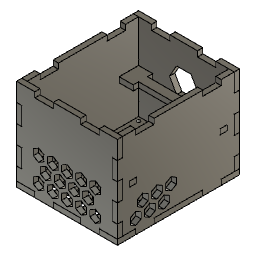
case (Autodesk Fusion 360 design; units mm, degrees)
Autodesk Fusion 360 part; units mm, degrees
(part 1 of 2)
ref_plane "WorkPlane4" through (0, 0, -25.9) normal (0, 0, 1) x (1, 0, 0)
sketch "Bottom" plane through (0, 0, -25.9) normal (0, 0, 1) x (1, 0, 0)
  line L0 (28.5, -34.5) -> (-28.5, -34.5)
  line L1 (-28.5, -34.5) -> (-28.5, 34.5)
  line L2 (-28.5, 34.5) -> (28.5, 34.5)
  line L3 (28.5, 34.5) -> (28.5, -34.5)
  line L4 (28.5, -34.5) -> (-28.5, 34.5) construction
  line L5 (-28.5, -34.5) -> (28.5, 34.5) construction
  line L6 (-18.14, 34.5) -> (-7.78, 34.5)
  line L7 (-7.78, 34.5) -> (-7.78, 31.5)
  line L8 (-7.78, 31.5) -> (-18.14, 31.5)
  line L9 (-18.14, 31.5) -> (-18.14, 34.5)
  line L10 (-28.5, 49.5405) -> (-18.14, 49.5405) construction
  line L11 (-28.5, 24.14) -> (-25.5, 24.14)
  line L12 (-25.5, 24.14) -> (-25.5, 13.78)
  line L13 (-25.5, 13.78) -> (-28.5, 13.78)
  line L14 (-28.5, 13.78) -> (-28.5, 24.14)
  line L15 (-32.8454, 24.14) -> (-32.8454, 34.5) construction
  line L16 (0, 34.5) -> (0, -34.5) construction
  line L17 (7.78, 34.5) -> (7.78, 31.5)
  line L18 (28.5, 49.5405) -> (18.14, 49.5405) construction
  line L19 (7.78, 31.5) -> (18.14, 31.5)
  line L20 (18.14, 31.5) -> (18.14, 34.5)
  line L21 (18.14, 34.5) -> (7.78, 34.5)
  line L22 (-28.5, 0) -> (28.5, 0) construction
  line L23 (-28.5, -24.14) -> (-25.5, -24.14)
  line L24 (-28.5, -13.78) -> (-28.5, -24.14)
  line L25 (-25.5, -24.14) -> (-25.5, -13.78)
  line L26 (-25.5, -13.78) -> (-28.5, -13.78)
  line L27 (-32.8454, -24.14) -> (-32.8454, -34.5) construction
  line L28 (28.5, 13.78) -> (28.5, 24.14)
  line L29 (28.5, -13.78) -> (28.5, -24.14)
  line L30 (25.5, 13.78) -> (28.5, 13.78)
  line L31 (28.5, 24.14) -> (25.5, 24.14)
  line L32 (32.8454, 24.14) -> (32.8454, 34.5) construction
  line L33 (28.5, -24.14) -> (25.5, -24.14)
  line L34 (25.5, -24.14) -> (25.5, -13.78)
  line L35 (32.8454, -24.14) -> (32.8454, -34.5) construction
  line L36 (25.5, -13.78) -> (28.5, -13.78)
  line L37 (25.5, 24.14) -> (25.5, 13.78)
  line L38 (-7.78, -31.5) -> (-18.14, -31.5)
  line L39 (7.78, -31.5) -> (18.14, -31.5)
  line L40 (18.14, -31.5) -> (18.14, -34.5)
  line L41 (18.14, -34.5) -> (7.78, -34.5)
  line L42 (-18.14, -34.5) -> (-7.78, -34.5)
  line L43 (28.5, -49.5405) -> (18.14, -49.5405) construction
  line L44 (7.78, -34.5) -> (7.78, -31.5)
  line L45 (-7.78, -34.5) -> (-7.78, -31.5)
  line L46 (-28.5, -49.5405) -> (-18.14, -49.5405) construction
  line L47 (-18.14, -31.5) -> (-18.14, -34.5)
  line L48 (-28.5, 34.5) -> (-23.32, 34.5) construction
  line L49 (-23.32, 34.5) -> (-23.32, 29.32) construction
  line L50 (-23.32, 29.32) -> (-28.5, 29.32) construction
  line L51 (-28.5, 29.32) -> (-28.5, 34.5) construction
  circle A0 centre (-23.32, 29.32) radius 1
  line L52 (-28.5, -34.5) -> (-23.32, -34.5) construction
  line L53 (-23.32, -34.5) -> (-23.32, -29.32) construction
  line L54 (-23.32, -29.32) -> (-28.5, -29.32) construction
  line L55 (-28.5, -29.32) -> (-28.5, -34.5) construction
  circle A1 centre (-23.32, -29.32) radius 1
  line L56 (28.5, -34.5) -> (23.32, -34.5) construction
  line L57 (23.32, -34.5) -> (23.32, -29.32) construction
  line L58 (23.32, -29.32) -> (28.5, -29.32) construction
  line L59 (28.5, -29.32) -> (28.5, -34.5) construction
  line L60 (28.5, 34.5) -> (23.32, 34.5) construction
  line L61 (23.32, 34.5) -> (23.32, 29.32) construction
  line L62 (23.32, 29.32) -> (28.5, 29.32) construction
  line L63 (28.5, 29.32) -> (28.5, 34.5) construction
  circle A2 centre (23.32, -29.32) radius 1
  circle A3 centre (23.32, 29.32) radius 1
  line L64 (0, -26.5) -> (-28.5, -26.5) construction
  line L65 (-13, -24.7679) -> (-16, -23.0359)
  line L66 (-1, -17.8397) -> (-4, -16.1077)
  line L67 (5, -24.7679) -> (5, -28.2321)
  line L68 (-3, -10.9115) -> (-3, -14.3756)
  line L69 (0, -26.5) -> (-1.5, -23.9019) construction
  line L70 (3, -28.2321) -> (3, -24.7679)
  line L71 (9, -21.3038) -> (12, -23.0359)
  line L72 (-11, -24.7679) -> (-11, -28.2321)
  line L73 (13, -14.3756) -> (16, -16.1077)
  line L74 (7, -21.3038) -> (7, -17.8397)
  line L75 (15, -21.3038) -> (15, -17.8397)
  line L76 (-16, -29.9641) -> (-13, -28.2321)
  line L77 (13, -28.2321) -> (16, -29.9641)
  line L78 (8, -9.1795) -> (5, -10.9115)
  line L79 (5, -14.3756) -> (8, -16.1077)
  line L80 (-19, -28.2321) -> (-16, -29.9641)
  line L81 (1, -17.8397) -> (1, -21.3038)
  line L82 (-13, -28.2321) -> (-13, -24.7679)
  line L83 (-13, -14.3756) -> (-13, -10.9115)
  line L84 (-11, -10.9115) -> (-11, -14.3756)
  line L85 (-4, -16.1077) -> (-7, -17.8397)
  line L86 (-5, -14.3756) -> (-5, -10.9115)
  line L87 (-8, -9.1795) -> (-11, -10.9115)
  line L88 (-3, -24.7679) -> (-3, -28.2321)
  line L89 (-8, -16.1077) -> (-5, -14.3756)
  line L90 (19, -28.2321) -> (19, -24.7679)
  line L91 (-19, -14.3756) -> (-16, -16.1077)
  line L92 (15, -17.8397) -> (12, -16.1077)
  line L93 (-19, -24.7679) -> (-19, -28.2321)
  line L94 (16, -29.9641) -> (19, -28.2321)
  line L95 (8, -29.9641) -> (11, -28.2321)
  line L96 (1, -21.3038) -> (4, -23.0359)
  line L97 (16, -16.1077) -> (19, -14.3756)
  line L98 (-12, -23.0359) -> (-9, -21.3038)
  line L99 (-4, -23.0359) -> (-1, -21.3038)
  line L100 (-11, -14.3756) -> (-8, -16.1077)
  line L101 (19, -14.3756) -> (19, -10.9115)
  line L102 (7, -17.8397) -> (4, -16.1077)
  line L103 (12, -16.1077) -> (9, -17.8397)
  line L104 (4, -23.0359) -> (7, -21.3038)
  line L105 (13, -10.9115) -> (13, -14.3756)
  line L106 (8, -23.0359) -> (5, -24.7679)
  line L107 (-5, -28.2321) -> (-5, -24.7679)
  line L108 (-16, -16.1077) -> (-13, -14.3756)
  line L109 (11, -14.3756) -> (11, -10.9115)
  line L110 (-7, -21.3038) -> (-4, -23.0359)
  line L111 (-5, -10.9115) -> (-8, -9.1795)
  line L112 (-3, -14.3756) -> (0, -16.1077)
  line L113 (-13, -10.9115) -> (-16, -9.1795)
  line L114 (3, -14.3756) -> (3, -10.9115)
  line L115 (-15, -21.3038) -> (-12, -23.0359)
  line L116 (-1, -21.3038) -> (-1, -17.8397)
  line L117 (19, -10.9115) -> (16, -9.1795)
  line L118 (-7, -17.8397) -> (-7, -21.3038)
  line L119 (0, -34.5) -> (0, -26.5) construction
  line L120 (-3, -28.2321) -> (0, -29.9641)
  line L121 (12, -23.0359) -> (15, -21.3038)
  line L122 (-15, -17.8397) -> (-15, -21.3038)
  line L123 (-28.5, -26.5) -> (-28.5, -34.5) construction
  line L124 (4, -16.1077) -> (1, -17.8397)
  line L125 (11, -28.2321) -> (11, -24.7679)
  line L126 (8, -16.1077) -> (11, -14.3756)
  line L127 (3, -10.9115) -> (0, -9.1795)
  line L128 (9, -17.8397) -> (9, -21.3038)
  line L129 (0, -23.0359) -> (-3, -24.7679)
  line L130 (16, -23.0359) -> (13, -24.7679)
  line L131 (0, -26.5) -> (3, -26.5) construction
  line L132 (0, -16.1077) -> (3, -14.3756)
  line L133 (0, -34.5) -> (0, 0) construction
  line L134 (-28.5, -34.5) -> (0, -34.5) construction
  line L135 (11, -10.9115) -> (8, -9.1795)
  line L136 (-28.5, -34.5) -> (0, -34.5) construction
  line L137 (0, -26.5) -> (1.5, -23.9019) construction
  line L138 (-16, -23.0359) -> (-19, -24.7679)
  line L139 (-12, -16.1077) -> (-15, -17.8397)
  line L140 (5, -28.2321) -> (8, -29.9641)
  line L141 (16, -9.1795) -> (13, -10.9115)
  line L142 (5, -10.9115) -> (5, -14.3756)
  line L143 (-16, -9.1795) -> (-19, -10.9115)
  line L144 (-11, -28.2321) -> (-8, -29.9641)
  line L145 (-28.5, 0) -> (-28.5, -34.5) construction
  line L146 (19, -24.7679) -> (16, -23.0359)
  line L147 (11, -24.7679) -> (8, -23.0359)
  line L148 (0, -9.1795) -> (-3, -10.9115)
  line L149 (-5, -24.7679) -> (-8, -23.0359)
  line L150 (-9, -17.8397) -> (-12, -16.1077)
  line L151 (0, -29.9641) -> (3, -28.2321)
  line L152 (-19, -10.9115) -> (-19, -14.3756)
  line L153 (-8, -23.0359) -> (-11, -24.7679)
  line L154 (-9, -21.3038) -> (-9, -17.8397)
  line L155 (-8, -29.9641) -> (-5, -28.2321)
  line L156 (13, -24.7679) -> (13, -28.2321)
  line L157 (3, -24.7679) -> (0, -23.0359)
  point P0 (30, -50)
  point P1 (28.5, 34.5)
  point P2 (32.8454, 34.5)
  point P3 (-28.5, -49.5405)
  point P4 (-28.5, -34.5)
  point P5 (28.5, 49.5405)
  point P6 (28.5, -34.5)
  point P7 (28.5, 34.5)
  point P8 (28.5, -34.5)
  point P9 (28.5, -49.5405)
  point P10 (28.5, 0)
  point P11 (28.5, -34.5)
  point P12 (0, -34.5)
  point P13 (-28.5, -34.5)
  point P14 (-32.8454, -34.5)
  point P15 (28.5, -34.5)
  point P16 (28.5, -49.5405)
  point P17 (28.5, -34.5)
  point P18 (0, -26.5)
  point P19 (0, -26.5)
  dimension "d32" = 57
  dimension "d33" = 69
  dimension "d34" = 10.36
  dimension "d35" = 3
  dimension "d36" = 10.36
  dimension "d37" = 3
  dimension "d38" = 10.36
  dimension "d39" = 10.36
  dimension "d326" = 5.18
  dimension "d327" = 5.18
  dimension "d328" = 2
  dimension "d329" = 5.18
  dimension "d330" = 5.18
  dimension "d331" = 2
  dimension "d332" = 5.18
  dimension "d333" = 5.18
  dimension "d334" = 5.18
  dimension "d335" = 5.18
  dimension "d336" = 2
  dimension "d337" = 2
  dimension "d384" = 8
  dimension "d385" = 0
  dimension "d388" = 8
  dimension "d389" = 0
  dimension "d392" = 8
  dimension "d393" = 0
  dimension "d396" = 8
  dimension "d397" = 0
  dimension "d398" = 28.5
  dimension "d399" = 34.5
  dimension "d400" = 28.5
  dimension "d401" = 8
  dimension "d402" = 3
  constraint horizontal L0
  constraint perpendicular L0 L1
  constraint parallel L0 L2
  constraint parallel L1 L3
  constraint coincident L4 L133.end
  constraint coincident L5 L133.end
  constraint coincident L133.end origin
  constraint horizontal L6
  constraint vertical L7
  constraint horizontal L8
  constraint vertical L9
  constraint coincident L2 L6.start
  constraint coincident L1 L10.start
  constraint coincident L9 L10.end
  constraint perpendicular L9 L10
  constraint horizontal L11
  constraint vertical L12
  constraint horizontal L13
  constraint vertical L14
  constraint coincident L1 L11.start
  constraint coincident L11 L15.start
  constraint coincident L2 L15.end
  constraint perpendicular L2 L15
  constraint midpoint L2 L16.start
  constraint midpoint L0 P12
  constraint symmetric L1.end L16 P7
  constraint symmetric L6.start L16 L20.end
  constraint symmetric L6.end L16 L17.start
  constraint symmetric L7.end L16 L17.end
  constraint symmetric L8.end L16 L19.end
  constraint symmetric L10.start L16 P5
  constraint symmetric L10.end L16 L18.end
  constraint symmetric L15.end L16 P2
  constraint midpoint L1 L22.start
  constraint midpoint L3 P10
  constraint symmetric L1.end L22 P13
  constraint symmetric L10.start L22 P3
  constraint symmetric L11.start L22 L23.start
  constraint symmetric L11.end L22 L23.end
  constraint symmetric L12.end L22 L25.end
  constraint symmetric L13.end L22 L24.start
  constraint symmetric L15.start L22 L27.start
  constraint symmetric L15.end L22 P14
  constraint symmetric P13 L16 P17
  constraint symmetric L11.start L16 L28.end
  constraint symmetric L11.end L16 L31.end
  constraint symmetric L12.end L16 L30.start
  constraint symmetric L13.end L16 L28.start
  constraint symmetric L15.start L16 L32.start
  constraint symmetric L16 L22.start P10
  constraint symmetric L16 L23.start L29.end
  constraint symmetric L16 L23.end L33.end
  constraint symmetric L16 P3 P16
  constraint symmetric L16 L25.end L34.end
  constraint symmetric L16 L27.start L35.start
  constraint symmetric L16 P14 L35.end
  constraint symmetric L16 L24.start L29.start
  constraint symmetric L16 P13 P17
  constraint symmetric P7 L22 P17
  constraint symmetric L6.start L22 L42.start
  constraint symmetric L6.end L22 L42.end
  constraint symmetric L7.end L22 L38.start
  constraint symmetric L8.end L22 L38.end
  constraint symmetric L10.end L22 L46.end
  constraint symmetric L16.start L22 P12
  constraint symmetric L17.end L22 L39.start
  constraint symmetric P5 L22 P16
  constraint symmetric L20.end L22 L40.end
  constraint symmetric L17.start L22 L41.end
  constraint symmetric L18.end L22 L43.end
  constraint symmetric L19.end L22 L39.end
  constraint symmetric L22 P5 P16
  constraint symmetric L22 P7 P17
  constraint horizontal L48
  constraint vertical L49
  constraint horizontal L50
  constraint vertical L51
  constraint coincident L49.end L50.start
  constraint horizontal L52
  constraint vertical L53
  constraint horizontal L54
  constraint vertical L55
  constraint coincident P13 P4
  constraint coincident L53.end L54.start
  constraint horizontal L56
  constraint vertical L57
  constraint horizontal L58
  constraint vertical L59
  constraint coincident P17 P15
  constraint horizontal L60
  constraint vertical L61
  constraint horizontal L62
  constraint vertical L63
  constraint coincident P7 P1
  constraint coincident L57.end L58.start
  constraint coincident L61.end L62.start
  constraint vertical L145
  constraint horizontal L136
  constraint vertical L133
  constraint horizontal L134
  constraint vertical L119
  constraint horizontal L64
  constraint vertical L123
  constraint coincident P19 P18
  constraint vertical L88
  constraint midpoint L137.end L157
  constraint midpoint L69.end L129
  constraint midpoint L131.end L70
  measures "d32" distance of L1.end P7
  measures "d33" distance of P13 L1.end
  measures "d34" distance of L6.start L6.end
  measures "d35" distance of L6.start L8.end
  measures "d36" distance of L10.start L10.end
  measures "d37" distance of L11.start L11.end
  measures "d38" distance of L11.start L13.end
  measures "d39" distance of L15.start L15.end
  measures "d326" distance of L1.end L48.end
  measures "d327" distance of L1.end L50.end
  measures "d328" diameter of A0
  measures "d329" distance of P13 L52.end
  measures "d330" distance of P13 L54.end
  measures "d331" diameter of A1
  measures "d332" distance of P17 L56.end
  measures "d333" distance of P17 L58.end
  measures "d334" distance of P7 L60.end
  measures "d335" distance of P7 L62.end
  measures "d336" diameter of A2
  measures "d337" diameter of A3
  measures "d398" distance of L133.end L22.start
  measures "d399" distance of L133.end P12
  measures "d400" distance of P13 P12
  measures "d401" distance of P13 L64.end
  measures "d402" distance of P19 L70
ref_plane "WorkPlane5" through (0, 34.5, 0) normal (0, 1, 0) x (0, 0, 1)
sketch "Back" plane through (0, 34.5, 0) normal (0, 1, 0) x (1, 0, 0)
  line L0 (28.5, 25.9) -> (-28.5, 25.9)
  line L1 (-28.5, 25.9) -> (-28.5, -25.9)
  line L2 (-28.5, -25.9) -> (28.5, -25.9)
  line L3 (28.5, -25.9) -> (28.5, 25.9)
  line L4 (28.5, 25.9) -> (-28.5, -25.9) construction
  line L5 (-28.5, 25.9) -> (28.5, -25.9) construction
  line L6 (28.5, -15.54) -> (25.5, -15.54)
  line L7 (25.5, -15.54) -> (25.5, -5.18)
  line L8 (25.5, -5.18) -> (28.5, -5.18)
  line L9 (28.5, -5.18) -> (28.5, -15.54)
  line L10 (27.7157, -25.9) -> (27.7157, -15.54) construction
  line L11 (-28.5, 0) -> (28.5, 0) construction
  line L12 (0, -25.9) -> (0, 25.9) construction
  line L13 (27.7157, 25.9) -> (27.7157, 15.54) construction
  line L14 (28.5, 5.18) -> (28.5, 15.54)
  line L15 (28.5, 15.54) -> (25.5, 15.54)
  line L16 (25.5, 5.18) -> (28.5, 5.18)
  line L17 (25.5, 15.54) -> (25.5, 5.18)
  line L18 (-27.7157, -25.9) -> (-27.7157, -15.54) construction
  line L19 (-28.5, -5.18) -> (-28.5, -15.54)
  line L20 (-28.5, -15.54) -> (-25.5, -15.54)
  line L21 (-25.5, -5.18) -> (-28.5, -5.18)
  line L22 (-25.5, -15.54) -> (-25.5, -5.18)
  line L23 (-28.5, 15.54) -> (-25.5, 15.54)
  line L24 (-25.5, 15.54) -> (-25.5, 5.18)
  line L25 (-28.5, 5.18) -> (-28.5, 15.54)
  line L26 (-25.5, 5.18) -> (-28.5, 5.18)
  line L27 (-27.7157, 25.9) -> (-27.7157, 15.54) construction
  line L28 (18.14, -25.9) -> (7.78, -25.9)
  line L29 (7.78, -25.9) -> (7.78, -22.9)
  line L30 (7.78, -22.9) -> (18.14, -22.9)
  line L31 (18.14, -22.9) -> (18.14, -25.9)
  line L32 (-7.78, -25.9) -> (-18.14, -25.9)
  line L33 (-18.14, -25.9) -> (-18.14, -22.9)
  line L34 (-18.14, -22.9) -> (-7.78, -22.9)
  line L35 (-7.78, -22.9) -> (-7.78, -25.9)
  line L36 (18.14, -24.4) -> (28.5, -24.4) construction
  line L37 (-18.14, -24.4) -> (-28.5, -24.4) construction
  line L38 (0, 0) -> (0, -5.6) construction
  line L39 (-8.0829, -5.6) -> (-4.0415, -12.6)
  line L40 (-4.0415, -12.6) -> (4.0415, -12.6)
  line L41 (4.0415, -12.6) -> (8.0829, -5.6)
  line L42 (8.0829, -5.6) -> (4.0415, 1.4)
  line L43 (4.0415, 1.4) -> (-4.0415, 1.4)
  line L44 (-4.0415, 1.4) -> (-8.0829, -5.6)
  point P0 (0, -5.6)
  dimension "d45" = 57
  dimension "d46" = 51.8
  dimension "d47" = 3
  dimension "d48" = 10.36
  dimension "d49" = 10.36
  dimension "d306" = 10.36
  dimension "d307" = 3
  dimension "d308" = 10.36
  dimension "d309" = 3
  dimension "d310" = 10.36
  dimension "d311" = 10.36
  dimension "d314" = 5.6
  dimension "d315" = 7
  constraint horizontal L0
  constraint perpendicular L0 L1
  constraint parallel L0 L2
  constraint parallel L1 L3
  constraint coincident L4 L38.start
  constraint coincident L5 L38.start
  constraint coincident L38.start origin
  constraint horizontal L6
  constraint vertical L7
  constraint horizontal L8
  constraint vertical L9
  constraint coincident L3 L6.start
  constraint coincident L2 L10.start
  constraint coincident L6 L10.end
  constraint perpendicular L6 L10
  constraint midpoint L1 L11.start
  constraint midpoint L3 L11.end
  constraint midpoint L2 L12.start
  constraint midpoint L0 L12.end
  constraint symmetric L6.start L11 L14.end
  constraint symmetric L6.end L11 L15.end
  constraint symmetric L7.end L11 L16.start
  constraint symmetric L8.end L11 L14.start
  constraint symmetric L10.start L11 L13.start
  constraint symmetric L10.end L11 L13.end
  constraint symmetric L6.start L12 L19.end
  constraint symmetric L6.end L12 L20.end
  constraint symmetric L7.end L12 L21.start
  constraint symmetric L8.end L12 L19.start
  constraint symmetric L10.start L12 L18.start
  constraint symmetric L10.end L12 L18.end
  constraint symmetric L12 L13.start L27.start
  constraint symmetric L12 L13.end L27.end
  constraint symmetric L12 L14.start L25.start
  constraint symmetric L12 L14.end L23.start
  constraint symmetric L12 L15.end L23.end
  constraint symmetric L12 L16.start L24.end
  constraint horizontal L28
  constraint vertical L29
  constraint horizontal L30
  constraint vertical L31
  constraint coincident L2 L28.start
  constraint horizontal L32
  constraint vertical L33
  constraint horizontal L34
  constraint vertical L35
  constraint coincident L2 L32.start
  constraint midpoint L31 L36.start
  constraint coincident L3 L36.end
  constraint perpendicular L3 L36
  constraint midpoint L33 L37.start
  constraint coincident L1 L37.end
  constraint perpendicular L1 L37
  constraint vertical L38
  constraint coincident P0 L38.end
  constraint horizontal L40
  measures "d45" distance of L1.end L2.end
  measures "d46" distance of L0.end L1.end
  measures "d47" distance of L6.start L6.end
  measures "d48" distance of L6.start L8.end
  measures "d49" distance of L10.start L10.end
  measures "d306" distance of L28.start L28.end
  measures "d307" distance of L28.start L30.end
  measures "d308" distance of L32.start L32.end
  measures "d309" distance of L32.start L34.end
  measures "d310" distance of L36.start L36.end
  measures "d311" distance of L37.start L37.end
  measures "d314" distance of L38.start P0
  measures "d315" distance of P0 L44
ref_plane "WorkPlane6" through (0, -34.5, 0) normal (0, 1, 0) x (0, 0, 1)
sketch "Front" plane through (0, -34.5, 0) normal (0, 1, 0) x (1, 0, 0)
  line L0 (28.5, 25.9) -> (-28.5, 25.9)
  line L1 (-28.5, 25.9) -> (-28.5, -25.9)
  line L2 (-28.5, -25.9) -> (28.5, -25.9)
  line L3 (28.5, -25.9) -> (28.5, 25.9)
  line L4 (28.5, 25.9) -> (-28.5, -25.9) construction
  line L5 (-28.5, 25.9) -> (28.5, -25.9) construction
  line L6 (-28.5, -15.54) -> (-25.5, -15.54)
  line L7 (-25.5, -15.54) -> (-25.5, -5.18)
  line L8 (-25.5, -5.18) -> (-28.5, -5.18)
  line L9 (-28.5, -5.18) -> (-28.5, -15.54)
  line L10 (0, -25.9) -> (0, 25.9) construction
  line L11 (-28.5, 0) -> (28.5, 0) construction
  line L12 (25.5, -15.54) -> (25.5, -5.18)
  line L13 (28.5, -15.54) -> (25.5, -15.54)
  line L14 (28.5, -5.18) -> (28.5, -15.54)
  line L15 (25.5, -5.18) -> (28.5, -5.18)
  line L16 (28.5, 15.54) -> (25.5, 15.54)
  line L17 (-28.5, 15.54) -> (-25.5, 15.54)
  line L18 (28.5, 5.18) -> (28.5, 15.54)
  line L19 (25.5, 5.18) -> (28.5, 5.18)
  line L20 (-25.5, 15.54) -> (-25.5, 5.18)
  line L21 (-28.5, 5.18) -> (-28.5, 15.54)
  line L22 (-25.5, 5.18) -> (-28.5, 5.18)
  line L23 (25.5, 15.54) -> (25.5, 5.18)
  line L24 (-27, -15.54) -> (-27, -25.9) construction
  line L25 (-18.14, -25.9) -> (-7.78, -25.9)
  line L26 (-7.78, -25.9) -> (-7.78, -22.9)
  line L27 (-7.78, -22.9) -> (-18.14, -22.9)
  line L28 (-18.14, -22.9) -> (-18.14, -25.9)
  line L29 (-18.14, -24.4) -> (-28.5, -24.4) construction
  line L30 (7.78, -25.9) -> (18.14, -25.9)
  line L31 (18.14, -25.9) -> (18.14, -22.9)
  line L32 (18.14, -22.9) -> (7.78, -22.9)
  line L33 (7.78, -22.9) -> (7.78, -25.9)
  line L34 (18.14, -24.4) -> (28.5, -24.4) construction
  line L35 (-15, 9.2397) -> (-12, 7.5077)
  line L36 (0, 7.5077) -> (-3, 5.7756)
  line L37 (0, 17.9) -> (-1.5, 15.3019) construction
  line L38 (-4, 14.4359) -> (-7, 12.7038)
  line L39 (0, 25.9) -> (0, 17.9) construction
  line L40 (-3, 16.1679) -> (0, 14.4359)
  line L41 (-1, 9.2397) -> (-1, 12.7038)
  line L42 (-5, 19.6321) -> (-8, 21.3641)
  line L43 (-11, 16.1679) -> (-8, 14.4359)
  line L44 (-8, 14.4359) -> (-5, 16.1679)
  line L45 (-8, 21.3641) -> (-11, 19.6321)
  line L46 (-3, 19.6321) -> (-3, 16.1679)
  line L47 (-16, 7.5077) -> (-19, 5.7756)
  line L48 (-5, 5.7756) -> (-8, 7.5077)
  line L49 (-5, 16.1679) -> (-5, 19.6321)
  line L50 (-3, 5.7756) -> (-3, 2.3115)
  line L51 (-13, 5.7756) -> (-16, 7.5077)
  line L52 (0, 17.9) -> (-28.5, 17.9) construction
  line L53 (-11, 5.7756) -> (-11, 2.3115)
  line L54 (-8, 7.5077) -> (-11, 5.7756)
  line L55 (0, 0) -> (-28.5, 0) construction
  line L56 (-13, 2.3115) -> (-13, 5.7756)
  line L57 (-28.5, 0) -> (-28.5, 25.9) construction
  line L58 (-4, 7.5077) -> (-1, 9.2397)
  line L59 (-7, 9.2397) -> (-4, 7.5077)
  line L60 (-3, 2.3115) -> (0, 0.5795)
  line L61 (0, 21.3641) -> (-3, 19.6321)
  line L62 (-8, 0.5795) -> (-5, 2.3115)
  line L63 (-28.5, 25.9) -> (0, 25.9) construction
  line L64 (-11, 19.6321) -> (-11, 16.1679)
  line L65 (-13, 19.6321) -> (-16, 21.3641)
  line L66 (-12, 14.4359) -> (-15, 12.7038)
  line L67 (-13, 16.1679) -> (-13, 19.6321)
  line L68 (-19, 5.7756) -> (-19, 2.3115)
  line L69 (-28.5, 25.9) -> (0, 25.9) construction
  line L70 (-16, 0.5795) -> (-13, 2.3115)
  line L71 (-5, 2.3115) -> (-5, 5.7756)
  line L72 (-19, 19.6321) -> (-19, 16.1679)
  line L73 (-28.5, 17.9) -> (-28.5, 25.9) construction
  line L74 (-11, 2.3115) -> (-8, 0.5795)
  line L75 (-12, 7.5077) -> (-9, 9.2397)
  line L76 (-1, 12.7038) -> (-4, 14.4359)
  line L77 (-19, 2.3115) -> (-16, 0.5795)
  line L78 (-15, 12.7038) -> (-15, 9.2397)
  line L79 (-16, 14.4359) -> (-13, 16.1679)
  line L80 (-16, 21.3641) -> (-19, 19.6321)
  line L81 (-19, 16.1679) -> (-16, 14.4359)
  line L82 (-9, 12.7038) -> (-12, 14.4359)
  line L83 (-7, 12.7038) -> (-7, 9.2397)
  line L84 (-9, 9.2397) -> (-9, 12.7038)
  line L85 (0, 25.9) -> (0, 0) construction
  line L86 (3, 5.7756) -> (0, 7.5077)
  line L87 (0, 0.5795) -> (3, 2.3115)
  line L88 (3, 19.6321) -> (0, 21.3641)
  line L89 (0, 14.4359) -> (3, 16.1679)
  line L90 (0, 17.9) -> (3, 17.9) construction
  line L91 (0, 17.9) -> (1.5, 15.3019) construction
  line L92 (9, 12.7038) -> (9, 9.2397)
  line L93 (1, 12.7038) -> (1, 9.2397)
  line L94 (7, 9.2397) -> (7, 12.7038)
  line L95 (15, 9.2397) -> (15, 12.7038)
  line L96 (4, 7.5077) -> (7, 9.2397)
  line L97 (11, 2.3115) -> (11, 5.7756)
  line L98 (5, 19.6321) -> (5, 16.1679)
  line L99 (19, 16.1679) -> (19, 19.6321)
  line L100 (13, 2.3115) -> (16, 0.5795)
  line L101 (16, 0.5795) -> (19, 2.3115)
  line L102 (4, 14.4359) -> (1, 12.7038)
  line L103 (12, 7.5077) -> (15, 9.2397)
  line L104 (19, 5.7756) -> (16, 7.5077)
  line L105 (13, 19.6321) -> (13, 16.1679)
  line L106 (5, 2.3115) -> (8, 0.5795)
  line L107 (15, 12.7038) -> (12, 14.4359)
  line L108 (1, 9.2397) -> (4, 7.5077)
  line L109 (9, 9.2397) -> (12, 7.5077)
  line L110 (3, 16.1679) -> (3, 19.6321)
  line L111 (11, 5.7756) -> (8, 7.5077)
  line L112 (16, 21.3641) -> (13, 19.6321)
  line L113 (13, 5.7756) -> (13, 2.3115)
  line L114 (8, 21.3641) -> (5, 19.6321)
  line L115 (19, 2.3115) -> (19, 5.7756)
  line L116 (13, 16.1679) -> (16, 14.4359)
  line L117 (11, 16.1679) -> (11, 19.6321)
  line L118 (19, 19.6321) -> (16, 21.3641)
  line L119 (16, 7.5077) -> (13, 5.7756)
  line L120 (12, 14.4359) -> (9, 12.7038)
  line L121 (3, 2.3115) -> (3, 5.7756)
  line L122 (8, 7.5077) -> (5, 5.7756)
  line L123 (5, 5.7756) -> (5, 2.3115)
  line L124 (8, 14.4359) -> (11, 16.1679)
  line L125 (8, 0.5795) -> (11, 2.3115)
  line L126 (16, 14.4359) -> (19, 16.1679)
  line L127 (11, 19.6321) -> (8, 21.3641)
  line L128 (7, 12.7038) -> (4, 14.4359)
  line L129 (5, 16.1679) -> (8, 14.4359)
  point P0 (30.1373, -20.0214)
  point P1 (30.1373, 20.0214)
  point P2 (0, 25.9)
  point P3 (28.5, 25.9)
  point P4 (-30, 20)
  point P5 (0, 17.9)
  dimension "d61" = 57
  dimension "d62" = 51.8
  dimension "d63" = 3
  dimension "d64" = 10.36
  dimension "d85" = 10.36
  dimension "d280" = 10.36
  dimension "d281" = 3
  dimension "d282" = 10.36
  dimension "d283" = 10.36
  dimension "d284" = 3
  dimension "d285" = 10.36
  dimension "d354" = 8
  dimension "d355" = 0
  dimension "d358" = 8
  dimension "d359" = 0
  dimension "d362" = 8
  dimension "d363" = 0
  dimension "d366" = 8
  dimension "d367" = 0
  dimension "d368" = 28.5
  dimension "d369" = 25.9
  dimension "d370" = 28.5
  dimension "d371" = 8
  dimension "d372" = 3
  constraint horizontal L0
  constraint perpendicular L0 L1
  constraint parallel L0 L2
  constraint parallel L1 L3
  constraint coincident L4 L55.start
  constraint coincident L5 L55.start
  constraint coincident L55.start L85.end
  constraint horizontal L6
  constraint vertical L7
  constraint horizontal L8
  constraint vertical L9
  constraint coincident L1 L6.start
  constraint midpoint L2 L10.start
  constraint midpoint L0 P2
  constraint midpoint L1 L11.start
  constraint midpoint L3 L11.end
  constraint symmetric L6.start L10 L13.start
  constraint symmetric L6.end L10 L12.start
  constraint symmetric L7.end L10 L12.end
  constraint symmetric L8.end L10 L14.start
  constraint symmetric L2.end L11 P3
  constraint symmetric L6.start L11 L17.start
  constraint symmetric L6.end L11 L17.end
  constraint symmetric L7.end L11 L20.end
  constraint symmetric L8.end L11 L21.start
  constraint symmetric L10.start L11 P2
  constraint symmetric L11 L12.end L19.start
  constraint symmetric L11 L14.start L18.start
  constraint symmetric L11 L13.start L16.start
  constraint symmetric L11 L12.start L16.end
  constraint symmetric L11 P0 P1
  constraint midpoint L6 L24.start
  constraint coincident L2 L24.end
  constraint perpendicular L2 L24
  constraint horizontal L25
  constraint vertical L26
  constraint horizontal L27
  constraint vertical L28
  constraint coincident L2 L25.start
  constraint midpoint L28 L29.start
  constraint coincident L1 L29.end
  constraint perpendicular L1 L29
  constraint horizontal L30
  constraint vertical L31
  constraint horizontal L32
  constraint vertical L33
  constraint coincident L2 L30.start
  constraint midpoint L31 L34.start
  constraint coincident L3 L34.end
  constraint perpendicular L3 L34
  constraint horizontal L55
  constraint vertical L57
  constraint horizontal L69
  constraint vertical L85
  constraint horizontal L63
  constraint vertical L39
  constraint horizontal L52
  constraint vertical L73
  constraint coincident P5 L37.start
  constraint midpoint L90.end L110
  constraint midpoint L91.end L89
  constraint midpoint L37.end L40
  constraint vertical L46
  measures "d61" distance of L1.end L2.end
  measures "d62" distance of L0.end L1.end
  measures "d63" distance of L6.start L6.end
  measures "d64" distance of L6.start L8.end
  measures "d85" distance of L24.start L24.end
  measures "d280" distance of L25.start L25.end
  measures "d281" distance of L25.start L27.end
  measures "d282" distance of L29.start L29.end
  measures "d283" distance of L30.start L30.end
  measures "d284" distance of L30.start L32.end
  measures "d285" distance of L34.start L34.end
  measures "d368" distance of L55.start L11.start
  measures "d369" distance of L55.start P2
  measures "d370" distance of P2 L0.end
  measures "d371" distance of L52.end L0.end
  measures "d372" distance of P5 L110
ref_plane "WorkPlane7" through (28.5, 0, 0) normal (1, 0, 0) x (0, 1, 0)
sketch "Right" plane through (28.5, 0, 0) normal (1, 0, 0) x (0, 1, 0)
  line L0 (34.5, -25.9) -> (-34.5, -25.9)
  line L1 (-34.5, -25.9) -> (-34.5, 25.9)
  line L2 (-34.5, 25.9) -> (34.5, 25.9)
  line L3 (34.5, 25.9) -> (34.5, -25.9)
  line L4 (34.5, -25.9) -> (-34.5, 25.9) construction
  line L5 (-34.5, -25.9) -> (34.5, 25.9) construction
  line L6 (-24.14, 25.9) -> (-13.78, 25.9)
  line L7 (-13.78, 25.9) -> (-13.78, 22.9)
  line L8 (-13.78, 22.9) -> (-24.14, 22.9)
  line L9 (-24.14, 22.9) -> (-24.14, 25.9)
  line L10 (-24.14, 24.4) -> (-34.5, 24.4) construction
  line L11 (13.78, 25.9) -> (24.14, 25.9)
  line L12 (24.14, 25.9) -> (24.14, 22.9)
  line L13 (24.14, 22.9) -> (13.78, 22.9)
  line L14 (13.78, 22.9) -> (13.78, 25.9)
  line L15 (24.14, 24.4) -> (34.5, 24.4) construction
  line L16 (-13.14, -19.6321) -> (-13.14, -16.1679)
  line L17 (-23.14, -9.2397) -> (-23.14, -12.7038)
  line L18 (-24.14, -14.4359) -> (-27.14, -16.1679)
  line L19 (-11.14, -16.1679) -> (-11.14, -19.6321)
  line L20 (-17.14, -12.7038) -> (-17.14, -9.2397)
  line L21 (-13.14, -16.1679) -> (-16.14, -14.4359)
  line L22 (-27.14, -16.1679) -> (-27.14, -19.6321)
  line L23 (-34.5, -25.9) -> (-24.14, -25.9) construction
  line L24 (-11.14, -19.6321) -> (-8.14, -21.3641)
  line L25 (-12.14, -7.5077) -> (-15.14, -9.2397)
  line L26 (-27.14, -19.6321) -> (-24.14, -21.3641)
  line L27 (-21.14, -16.1679) -> (-24.14, -14.4359)
  line L28 (-5.14, -16.1679) -> (-8.14, -14.4359)
  line L29 (-1.14, -9.2397) -> (-4.14, -7.5077)
  line L30 (-7.14, -12.7038) -> (-4.14, -14.4359)
  line L31 (-34.5, -25.9) -> (0, -25.9) construction
  line L32 (-34.5, 0) -> (-34.5, -25.9) construction
  line L33 (-1.14, -12.7038) -> (-1.14, -9.2397)
  line L34 (0, -25.9) -> (0, 0) construction
  line L35 (-4.14, -7.5077) -> (-7.14, -9.2397)
  line L36 (-8.14, -21.3641) -> (-5.14, -19.6321)
  line L37 (-5.14, -19.6321) -> (-5.14, -16.1679)
  line L38 (-7.14, -9.2397) -> (-7.14, -12.7038)
  line L39 (0, 0) -> (-34.5, 0) construction
  line L40 (-4.14, -14.4359) -> (-1.14, -12.7038)
  line L41 (-24.14, -21.3641) -> (-21.14, -19.6321)
  line L42 (-24.14, -17.9) -> (-22.64, -15.3019) construction
  line L43 (-15.14, -12.7038) -> (-12.14, -14.4359)
  line L44 (-24.14, -17.9) -> (-34.5, -17.9) construction
  line L45 (-9.14, -9.2397) -> (-12.14, -7.5077)
  line L46 (-9.14, -12.7038) -> (-9.14, -9.2397)
  line L47 (-24.14, -25.9) -> (-24.14, -17.9) construction
  line L48 (-21.14, -19.6321) -> (-21.14, -16.1679)
  line L49 (-23.14, -12.7038) -> (-20.14, -14.4359)
  line L50 (-19.14, -19.6321) -> (-16.14, -21.3641)
  line L51 (-24.14, -17.9) -> (-21.14, -17.9) construction
  line L52 (-34.5, -17.9) -> (-34.5, -25.9) construction
  line L53 (-8.14, -14.4359) -> (-11.14, -16.1679)
  line L54 (-12.14, -14.4359) -> (-9.14, -12.7038)
  line L55 (-16.14, -21.3641) -> (-13.14, -19.6321)
  line L56 (-16.14, -14.4359) -> (-19.14, -16.1679)
  line L57 (-20.14, -14.4359) -> (-17.14, -12.7038)
  line L58 (-19.14, -16.1679) -> (-19.14, -19.6321)
  line L59 (-17.14, -9.2397) -> (-20.14, -7.5077)
  line L60 (-20.14, -7.5077) -> (-23.14, -9.2397)
  line L61 (-15.14, -9.2397) -> (-15.14, -12.7038)
  point P0 (-24.14, -17.9)
  dimension "d74" = 69
  dimension "d75" = 51.8
  dimension "d288" = 10.36
  dimension "d289" = 3
  dimension "d290" = 10.36
  dimension "d291" = 10.36
  dimension "d292" = 3
  dimension "d293" = 10.36
  dimension "d375" = 8
  dimension "d376" = 8
  dimension "d377" = 34.5
  dimension "d378" = 25.9
  dimension "d379" = 10.36
  dimension "d380" = 8
  dimension "d381" = 3
  constraint horizontal L0
  constraint perpendicular L0 L1
  constraint parallel L0 L2
  constraint parallel L1 L3
  constraint coincident L4 L34.end
  constraint coincident L5 L34.end
  constraint coincident L34.end L39.start
  constraint horizontal L6
  constraint vertical L7
  constraint horizontal L8
  constraint vertical L9
  constraint coincident L2 L6.start
  constraint midpoint L9 L10.start
  constraint coincident L1 L10.end
  constraint perpendicular L1 L10
  constraint horizontal L11
  constraint vertical L12
  constraint horizontal L13
  constraint vertical L14
  constraint coincident L2 L11.start
  constraint midpoint L12 L15.start
  constraint coincident L3 L15.end
  constraint perpendicular L3 L15
  constraint horizontal L39
  constraint vertical L32
  constraint horizontal L31
  constraint vertical L34
  constraint horizontal L23
  constraint vertical L47
  constraint horizontal L44
  constraint vertical L52
  constraint coincident P0 L42.start
  constraint vertical L22
  constraint midpoint L42.end L27
  constraint midpoint L51.end L48
  measures "d74" distance of L1.end L2.end
  measures "d75" distance of L0.end L1.end
  measures "d288" distance of L6.start L6.end
  measures "d289" distance of L6.start L8.end
  measures "d290" distance of L10.start L10.end
  measures "d291" distance of L11.start L11.end
  measures "d292" distance of L11.start L13.end
  measures "d293" distance of L15.start L15.end
  measures "d377" distance of L32.start L34.end
  measures "d378" distance of L31.end L34.end
  measures "d379" distance of L23.end L0.end
  measures "d380" distance of L44.end L0.end
  measures "d381" distance of P0 L48
mirror "Mirror1" [no effect]
ref_plane "WorkPlane9" through (0, 0, -0.9) normal (0, 0, 1) x (1, 0, 0)
sketch "BackSupport" plane through (0, 0, -0.9) normal (0, 0, 1) x (1, 0, 0)
  line L0 (0, 0) -> (-25.5, 0) construction
  line L1 (-25.5, 0) -> (-25.5, 31.5) construction
  line L2 (-25.5, 31.5) -> (0, 31.5) construction
  line L3 (0, 31.5) -> (0, 0) construction
  line L4 (-25.5, 31.5) -> (-21.5, 31.5) construction
  line L5 (-21.5, 31.5) -> (-17.5, 31.5)
  line L6 (-17.5, 31.5) -> (-17.5, 34.5)
  line L7 (-17.5, 34.5) -> (-21.5, 34.5)
  line L8 (-21.5, 34.5) -> (-21.5, 31.5)
  line L9 (-25.5, 31.5) -> (-25.5, 27.5) construction
  line L10 (-25.5, 27.5) -> (-28.5, 27.5)
  line L11 (-28.5, 27.5) -> (-28.5, 23.5)
  line L12 (-28.5, 23.5) -> (-25.5, 23.5)
  line L13 (-25.5, 23.5) -> (-25.5, 27.5)
  line L14 (-25.5, 31.5) -> (-17.5, 31.5)
  line L15 (-17.5, 31.5) -> (-17.5, 20.5)
  line L16 (-17.5, 20.5) -> (-25.5, 20.5)
  line L17 (-25.5, 20.5) -> (-25.5, 31.5)
  line L18 (-17.5, 28.5) -> (0, 28.5)
  line L19 (0, 28.5) -> (0, 23.5)
  line L20 (0, 23.5) -> (-17.5, 23.5)
  line L21 (-17.5, 23.5) -> (-17.5, 28.5)
  line L22 (17.5, 28.5) -> (0, 28.5)
  line L23 (0, 28.5) -> (0, 23.5)
  line L24 (17.5, 23.5) -> (17.5, 28.5)
  line L25 (0, 23.5) -> (17.5, 23.5)
  line L26 (25.5, 31.5) -> (17.5, 31.5)
  line L27 (17.5, 31.5) -> (17.5, 20.5)
  line L28 (25.5, 20.5) -> (25.5, 31.5)
  line L29 (17.5, 20.5) -> (25.5, 20.5)
  line L30 (25.5, 27.5) -> (28.5, 27.5)
  line L31 (28.5, 27.5) -> (28.5, 23.5)
  line L32 (25.5, 23.5) -> (25.5, 27.5)
  line L33 (28.5, 23.5) -> (25.5, 23.5)
  line L34 (21.5, 31.5) -> (17.5, 31.5)
  line L35 (17.5, 31.5) -> (17.5, 34.5)
  line L36 (21.5, 34.5) -> (21.5, 31.5)
  line L37 (17.5, 34.5) -> (21.5, 34.5)
  line L38 (-17.5, 31.5) -> (-17.5, 28.5) construction
  dimension "d83" = 25.5
  dimension "d84" = 31.5
  dimension "d86" = 4
  dimension "d87" = 4
  dimension "d88" = 3
  dimension "d89" = 4
  dimension "d90" = 3
  dimension "d91" = 4
  dimension "d94" = 8
  dimension "d95" = 11
  dimension "d97" = 17.5
  dimension "d98" = 5
  dimension "d102" = 3
  constraint horizontal L0
  constraint vertical L1
  constraint horizontal L2
  constraint vertical L3
  constraint coincident L0.start L3.end
  constraint perpendicular L1 L4
  constraint horizontal L5
  constraint vertical L6
  constraint horizontal L7
  constraint vertical L8
  constraint perpendicular L2 L9
  constraint horizontal L10
  constraint vertical L11
  constraint horizontal L12
  constraint vertical L13
  constraint horizontal L14
  constraint vertical L15
  constraint horizontal L16
  constraint vertical L17
  constraint coincident L15 L18.start
  constraint horizontal L18
  constraint vertical L19
  constraint horizontal L20
  constraint vertical L21
  constraint symmetric L1.end L3 L26.start
  constraint symmetric L3 L4.end L34.start
  constraint symmetric L3 L5.end L26.end
  constraint symmetric L3 L6.end L35.end
  constraint symmetric L3 L7.end L36.start
  constraint symmetric L3 L9.end L30.start
  constraint symmetric L3 L10.end L30.end
  constraint symmetric L3 L11.end L31.end
  constraint symmetric L3 L12.end L32.start
  constraint symmetric L3 L15.end L27.end
  constraint symmetric L3 L16.end L28.start
  constraint symmetric L3 L18.start L22.start
  constraint symmetric L3 L18.end L19.start
  constraint symmetric L3 L19.end L20.start
  constraint symmetric L3 L20.end L24.start
  measures "d83" distance of L0.start L0.end
  measures "d84" distance of L0.start L2.end
  measures "d86" distance of L1.end L4.end
  measures "d87" distance of L4.end L5.end
  measures "d88" distance of L4.end L7.end
  measures "d89" distance of L1.end L9.end
  measures "d90" distance of L9.end L10.end
  measures "d91" distance of L9.end L12.end
  measures "d94" distance of L1.end L5.end
  measures "d95" distance of L1.end L16.end
  measures "d97" distance of L18.start L18.end
  measures "d98" distance of L18.start L20.end
  measures "d102" distance of L5.end L18.start
combine "Combine7" [no effect]
sketch "FrontSupport" plane through (0, 0, -0.9) normal (0, 0, 1) x (1, 0, 0)
  line L0 (0, 0) -> (-25.5, 0) construction
  line L1 (-25.5, 0) -> (-25.5, -31.5) construction
  line L2 (-25.5, -31.5) -> (0, -31.5) construction
  line L3 (0, -31.5) -> (0, 0) construction
  line L4 (-25.5, -31.5) -> (-21.5, -31.5) construction
  line L5 (-25.5, -31.5) -> (-25.5, -27.5) construction
  line L6 (-25.5, -27.5) -> (-28.5, -27.5)
  line L7 (-28.5, -27.5) -> (-28.5, -23.5)
  line L8 (-28.5, -23.5) -> (-25.5, -23.5)
  line L9 (-25.5, -23.5) -> (-25.5, -27.5)
  line L10 (-25.5, -31.5) -> (-17.5, -31.5)
  line L11 (-17.5, -31.5) -> (-17.5, -23.5)
  line L12 (-17.5, -23.5) -> (-25.5, -23.5)
  line L13 (-25.5, -23.5) -> (-25.5, -31.5)
  line L14 (25.5, -27.5) -> (28.5, -27.5)
  line L15 (28.5, -27.5) -> (28.5, -23.5)
  line L16 (28.5, -23.5) -> (25.5, -23.5)
  line L17 (25.5, -23.5) -> (25.5, -27.5)
  line L18 (0, 0) -> (25.5, 0) construction
  line L19 (25.5, 0) -> (25.5, -31.5) construction
  line L20 (25.5, -31.5) -> (0, -31.5) construction
  line L21 (0, -31.5) -> (0, 0) construction
  line L22 (25.5, -31.5) -> (22.5, -31.5)
  line L23 (22.5, -31.5) -> (22.5, -23.5)
  line L24 (22.5, -23.5) -> (25.5, -23.5)
  line L25 (25.5, -23.5) -> (25.5, -31.5)
  line L26 (25.5, -31.5) -> (0, -31.5)
  line L27 (0, -31.5) -> (0, -28.5)
  line L28 (0, -28.5) -> (25.5, -28.5)
  line L29 (25.5, -28.5) -> (25.5, -31.5)
  line L30 (0, -31.5) -> (-17.5, -31.5)
  line L31 (-17.5, -31.5) -> (-17.5, -28.5)
  line L32 (-17.5, -28.5) -> (0, -28.5)
  line L33 (0, -28.5) -> (0, -31.5)
  dimension "d103" = 25.5
  dimension "d104" = 31.5
  dimension "d105" = 4
  dimension "d108" = 4
  dimension "d109" = 3
  dimension "d110" = 4
  dimension "d112" = 8
  dimension "d113" = 8
  dimension "d114" = 25.5
  dimension "d115" = 31.5
  dimension "d116" = 3
  dimension "d117" = 8
  dimension "d118" = 25.5
  dimension "d119" = 3
  dimension "d120" = 17.5
  dimension "d121" = 3
  constraint horizontal L0
  constraint vertical L1
  constraint horizontal L2
  constraint vertical L3
  constraint coincident L0.start L3.end
  constraint perpendicular L1 L4
  constraint perpendicular L4 L5
  constraint horizontal L6
  constraint vertical L7
  constraint horizontal L8
  constraint vertical L9
  constraint horizontal L10
  constraint vertical L11
  constraint horizontal L12
  constraint vertical L13
  constraint symmetric L3 L5.end L14.start
  constraint symmetric L3 L6.end L14.end
  constraint symmetric L3 L7.end L15.end
  constraint symmetric L3 L8.end L16.end
  constraint horizontal L18
  constraint vertical L19
  constraint horizontal L20
  constraint vertical L21
  constraint horizontal L22
  constraint vertical L23
  constraint horizontal L24
  constraint vertical L25
  constraint horizontal L26
  constraint vertical L27
  constraint horizontal L28
  constraint vertical L29
  constraint horizontal L30
  constraint vertical L31
  constraint horizontal L32
  constraint vertical L33
  measures "d103" distance of L0.start L0.end
  measures "d104" distance of L0.start L2.end
  measures "d105" distance of L1.end L4.end
  measures "d108" distance of L1.end L5.end
  measures "d109" distance of L5.end L6.end
  measures "d110" distance of L5.end L8.end
  measures "d112" distance of L1.end L10.end
  measures "d113" distance of L1.end L8.end
  measures "d114" distance of L0.start L18.end
  measures "d115" distance of L0.start L2.end
  measures "d116" distance of L19.end L22.end
  measures "d117" distance of L19.end L16.end
  measures "d118" distance of L19.end L2.end
  measures "d119" distance of L19.end L28.end
  measures "d120" distance of L2.end L10.end
  measures "d121" distance of L2.end L27.end
combine "Combine10" [no effect]
ref_plane "WorkPlane10" through (-28.5, 0, 0) normal (1, 0, 0) x (0, 1, 0)
sketch "Left" plane through (-28.5, 0, 0) normal (1, 0, 0) x (0, 1, 0)
  line L0 (0, 0) -> (-34.5, 0) construction
  line L1 (-34.5, 0) -> (-34.5, -25.9) construction
  line L2 (-34.5, -25.9) -> (0, -25.9) construction
  line L3 (0, -25.9) -> (0, 0) construction
  line L4 (-34.5, -25.9) -> (-24.14, -25.9) construction
  line L5 (-24.14, -25.9) -> (-24.14, -17.9) construction
  line L6 (-24.14, -17.9) -> (-34.5, -17.9) construction
  line L7 (-34.5, -17.9) -> (-34.5, -25.9) construction
  line L8 (-27.14, -19.6321) -> (-24.14, -21.3641)
  line L9 (-24.14, -21.3641) -> (-21.14, -19.6321)
  line L10 (-21.14, -19.6321) -> (-21.14, -16.1679)
  line L11 (-21.14, -16.1679) -> (-24.14, -14.4359)
  line L12 (-24.14, -14.4359) -> (-27.14, -16.1679)
  line L13 (-27.14, -16.1679) -> (-27.14, -19.6321)
  line L14 (-24.14, -17.9) -> (-22.64, -15.3019) construction
  line L15 (-24.14, -17.9) -> (-21.14, -17.9) construction
  line L16 (-19.14, -19.6321) -> (-16.14, -21.3641)
  line L17 (-16.14, -21.3641) -> (-13.14, -19.6321)
  line L18 (-13.14, -19.6321) -> (-13.14, -16.1679)
  line L19 (-13.14, -16.1679) -> (-16.14, -14.4359)
  line L20 (-16.14, -14.4359) -> (-19.14, -16.1679)
  line L21 (-19.14, -16.1679) -> (-19.14, -19.6321)
  line L22 (-11.14, -19.6321) -> (-8.14, -21.3641)
  line L23 (-8.14, -21.3641) -> (-5.14, -19.6321)
  line L24 (-5.14, -19.6321) -> (-5.14, -16.1679)
  line L25 (-5.14, -16.1679) -> (-8.14, -14.4359)
  line L26 (-8.14, -14.4359) -> (-11.14, -16.1679)
  line L27 (-11.14, -16.1679) -> (-11.14, -19.6321)
  line L28 (-23.14, -12.7038) -> (-20.14, -14.4359)
  line L29 (-20.14, -14.4359) -> (-17.14, -12.7038)
  line L30 (-17.14, -12.7038) -> (-17.14, -9.2397)
  line L31 (-17.14, -9.2397) -> (-20.14, -7.5077)
  line L32 (-20.14, -7.5077) -> (-23.14, -9.2397)
  line L33 (-23.14, -9.2397) -> (-23.14, -12.7038)
  line L34 (-15.14, -12.7038) -> (-12.14, -14.4359)
  line L35 (-12.14, -14.4359) -> (-9.14, -12.7038)
  line L36 (-9.14, -12.7038) -> (-9.14, -9.2397)
  line L37 (-9.14, -9.2397) -> (-12.14, -7.5077)
  line L38 (-15.14, -9.2397) -> (-15.14, -12.7038)
  line L39 (-12.14, -7.5077) -> (-15.14, -9.2397)
  line L40 (-7.14, -12.7038) -> (-4.14, -14.4359)
  line L41 (-4.14, -14.4359) -> (-1.14, -12.7038)
  line L42 (-1.14, -12.7038) -> (-1.14, -9.2397)
  line L43 (-1.14, -9.2397) -> (-4.14, -7.5077)
  line L44 (-7.14, -9.2397) -> (-7.14, -12.7038)
  line L45 (-4.14, -7.5077) -> (-7.14, -9.2397)
  line L46 (-34.5, 25.9) -> (34.5, 25.9)
  line L47 (34.5, 25.9) -> (34.5, -25.9)
  line L48 (34.5, -25.9) -> (-34.5, -25.9)
  line L49 (-34.5, -25.9) -> (-34.5, 25.9)
  line L50 (-34.5, 25.9) -> (34.5, -25.9) construction
  line L51 (34.5, 25.9) -> (-34.5, -25.9) construction
  line L52 (24.14, 25.9) -> (13.78, 25.9)
  line L53 (13.78, 25.9) -> (13.78, 22.9)
  line L54 (13.78, 22.9) -> (24.14, 22.9)
  line L55 (24.14, 22.9) -> (24.14, 25.9)
  line L56 (-13.78, 25.9) -> (-24.14, 25.9)
  line L57 (-24.14, 25.9) -> (-24.14, 22.9)
  line L58 (-24.14, 22.9) -> (-13.78, 22.9)
  line L59 (-13.78, 22.9) -> (-13.78, 25.9)
  line L60 (24.14, 24.4) -> (34.5, 24.4) construction
  line L61 (-24.14, 24.4) -> (-34.5, 24.4) construction
  point P0 (-24.14, -17.9)
  dimension "d243" = 34.5
  dimension "d244" = 25.9
  dimension "d245" = 10.36
  dimension "d246" = 8
  dimension "d247" = 3
  dimension "d250" = 8
  dimension "d251" = 0
  dimension "d254" = 8
  dimension "d255" = 0
  dimension "d296" = 69
  dimension "d297" = 51.8
  dimension "d298" = 10.36
  dimension "d299" = 3
  dimension "d300" = 10.36
  dimension "d301" = 3
  dimension "d302" = 10.36
  dimension "d303" = 10.36
  constraint horizontal L0
  constraint vertical L1
  constraint horizontal L2
  constraint vertical L3
  constraint coincident L0.start L3.end
  constraint horizontal L4
  constraint vertical L5
  constraint horizontal L6
  constraint vertical L7
  constraint coincident P0 L5.end
  constraint vertical L10
  constraint midpoint L11 L14.end
  constraint midpoint L10 L15.end
  constraint horizontal L46
  constraint perpendicular L46 L47
  constraint parallel L46 L48
  constraint parallel L47 L49
  constraint coincident L50 L0.start
  constraint coincident L51 L0.start
  constraint horizontal L52
  constraint vertical L53
  constraint horizontal L54
  constraint vertical L55
  constraint coincident L46 L52.start
  constraint horizontal L56
  constraint vertical L57
  constraint horizontal L58
  constraint vertical L59
  constraint coincident L46 L56.start
  constraint midpoint L55 L60.start
  constraint coincident L47 L60.end
  constraint perpendicular L47 L60
  constraint midpoint L57 L61.start
  constraint coincident L49 L61.end
  constraint perpendicular L49 L61
  measures "d243" distance of L0.start L0.end
  measures "d244" distance of L0.start L2.end
  measures "d245" distance of L1.end L4.end
  measures "d246" distance of L1.end L6.end
  measures "d247" distance of P0 L13
  measures "d296" distance of L47.end L1.end
  measures "d297" distance of L46.end L47.end
  measures "d298" distance of L52.start L52.end
  measures "d299" distance of L52.start L54.end
  measures "d300" distance of L56.start L56.end
  measures "d301" distance of L56.start L58.end
  measures "d302" distance of L60.start L60.end
  measures "d303" distance of L61.start L61.end
extrude "Extrude15" cut sketch "Left" along normal blind 3 contours L8 L9 L10 L11 L12 L13 | L16 L17 L18 L19 L20 L21 | L22 L23 L24 L25 L26 L27 | L28 L29 L30 L31 L32 L33 | L34 L35 L36 L37 L38 L39 | L40 L41 L42 L43 L44 L45
ref_plane "WorkPlane11" through (0, 0, 25.9) normal (0, 0, 1) x (1, 0, 0)
sketch "Top" plane through (0, 0, 25.9) normal (0, 0, 1) x (1, 0, 0)
  line L0 (28.5, -34.5) -> (-28.5, -34.5)
  line L1 (-28.5, -34.5) -> (-28.5, 34.5)
  line L2 (-28.5, 34.5) -> (28.5, 34.5)
  line L3 (28.5, 34.5) -> (28.5, -34.5)
  line L4 (28.5, -34.5) -> (-28.5, 34.5) construction
  line L5 (-28.5, -34.5) -> (28.5, 34.5) construction
  line L6 (0, 0) -> (-28.5, 0) construction
  line L7 (-28.5, 0) -> (-28.5, 34.5) construction
  line L8 (-28.5, 34.5) -> (0, 34.5) construction
  line L9 (0, 34.5) -> (0, 0) construction
  line L10 (-28.5, 34.5) -> (0, 34.5) construction
  line L11 (0, 34.5) -> (0, 4.5) construction
  line L12 (0, 4.5) -> (-28.5, 4.5) construction
  line L13 (-28.5, 4.5) -> (-28.5, 34.5) construction
  line L14 (8, -2) -> (-8, -2)
  line L15 (-8, -2) -> (-8, 11)
  line L16 (-8, 11) -> (8, 11)
  line L17 (8, 11) -> (8, -2)
  line L18 (8, -2) -> (-8, 11) construction
  line L19 (-8, -2) -> (8, 11) construction
  point P0 (0, 4.5)
  dimension "d278" = 57
  dimension "d279" = 69
  dimension "d318" = 28.5
  dimension "d319" = 34.5
  dimension "d320" = 28.5
  dimension "d321" = 30
  dimension "d322" = 16
  dimension "d323" = 13
  constraint horizontal L0
  constraint perpendicular L0 L1
  constraint parallel L0 L2
  constraint parallel L1 L3
  constraint coincident L4 L6.start
  constraint coincident L5 L6.start
  constraint coincident L6.start L9.end
  constraint horizontal L6
  constraint vertical L7
  constraint horizontal L8
  constraint vertical L9
  constraint horizontal L10
  constraint vertical L11
  constraint horizontal L12
  constraint vertical L13
  constraint horizontal L14
  constraint perpendicular L14 L15
  constraint parallel L14 L16
  constraint parallel L15 L17
  constraint coincident L18 P0
  constraint coincident L19 P0
  constraint coincident P0 L11.end
  measures "d278" distance of L1.end L2.end
  measures "d279" distance of L0.end L1.end
  measures "d318" distance of L6.start L6.end
  measures "d319" distance of L6.start L8.end
  measures "d320" distance of L1.end L8.end
  measures "d321" distance of L1.end L12.end
  measures "d322" distance of L15.end L16.end
  measures "d323" distance of L14.end L15.end
extrude "Extrude19" cut sketch "Left" along normal blind 3 contours L46 L56 L57 L58 L59 | L46 L52 L53 L54 L55
extrude "Extrude26" add sketch "Front" along normal blind 3 separate body contours L0 L1 L2 L3 L6 L7 L8 L12 L13 L15 L16 L17 L19 L20 L22 L23 L26 L27 L28 L31 L32 L33 makes body 1